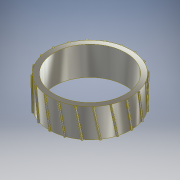
# Autodesk Inventor part: net
Saved by Autodesk Inventor 2018 (Build 220112000, 112)
## iProperties
Created: 2019-09-09
Part Number: net
Material: Silver
Document SubType Name: Modeling
Designer: dsikar
Density: 10.49 g/cm^3
Appearance: Silver
Author: dsikar
Autodesk Inventor part; units mm, degrees
ref_plane "YZ Plane" through (0, 0, 0) normal (1, 0, 0) x (0, 1, 0)
ref_plane "XY Plane" through (0, 0, 0) normal (0, 0, 1) x (1, 0, 0)
sketch "Sketch1" plane through (0, 0, 0) normal (0, 1, 0) x (-1, 0, 0)
  line L0 (8.7, 0) -> (9.9, 0)
  line L1 (9.9, 0) -> (9.9, 7)
  line L2 (9.9, 7) -> (8.7, 7)
  line L3 (8.7, 7) -> (8.7, 0)
  line L4 (0, -1.4) -> (0, 8.4) projected
  point P0 (0, 0)
  dimension "d0" = 1.2
  dimension "d1" = 7
  dimension "d2" = 8.7
  constraints: 8 end point, 2 parallel, 1 horizontal, 1 perpendicular
  measures "d0" distance of L2.end L1.end
  measures "d1" distance of L1.end L0.end
  measures "d2" distance from line of L3 point (0, 0)
revolve "Revolution1" add sketch "Sketch1" angle 360 about axis through (0, 0, -10) along (0, 0, 1)
ref_plane "Work Plane1" through (0, -15.5, 0) normal (0, 1, 0) x (-1, 0, 0)
sketch "Sketch8" plane through (0, -15.5, 0) normal (0, 1, 0) x (-1, 0, 0)
  line L0 (0, 0) -> (1.2343, 7)
  line L1 (0, 0) -> (7.8694, 0) construction
  line L2 (0.8281, 7) -> (-0.4062, 0)
  line L3 (1.2316, 6.985) -> (0.8281, 7)
  line L4 (-9.9, 7) -> (9.9, 7) projected
  line L5 (0, 0) -> (-0.4062, 0)
  line L6 (-9.9, 0) -> (9.9, 0) projected
  dimension "d19" = 80
  dimension "d20" = 0.4
  constraints: 10 end point, 4 point on line, 1 horizontal
  measures "d19" angle of L1 L0
  measures "d20" distance between parallel lines of L0 L2
emboss "Emboss3" sketch "Sketch8" operation add depth 0.3 direction (0, -1, 0) wrap yes faces at (-9.7718, 1.5881, 2.3333) contours L5 L2 L3 L0
fillet "Fillet2" radius 0.2 1 edges at (-0.2174, -10.1977, 3.5)
fillet "Fillet3" radius 0.2 1 edges at (-0.6341, -10.1803, 3.4925)
pattern_circular "Circular Pattern3" count 20 over 360 about axis through (0, 0, 3.5) along (0, 0, -1) of "Emboss3", "Fillet2", "Fillet3"
body "Solid1"
